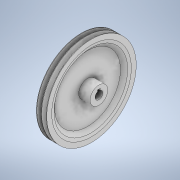
# Autodesk Inventor part: polia final
Saved by Autodesk Inventor 2022.1 (Build 261234020, 234B)
## iProperties
Created: 2023-10-20
Part Number: polia final
Material: Generic
Document SubType Name: Modeling
Designer: SENAI
Density: 1 g/cm^3
Appearance: Default
Author: SENAI
Autodesk Inventor part; units mm, degrees
ref_plane "YZ Plane" through (0, 0, 0) normal (1, 0, 0) x (0, 1, 0)
ref_plane "XZ Plane" through (0, 0, 0) normal (0, 1, 0) x (-1, 0, 0)
ref_plane "XY Plane" through (0, 0, 0) normal (0, 0, 1) x (1, 0, 0)
sketch "Sketch1" plane through (0, 0, 0) normal (0, 0, 1) x (1, 0, 0)
  line L0 (0, 0) -> (47, 0)
  line L1 (47, 10.25) -> (0, 10.25)
  line L2 (0, 10.25) -> (0, 17.75)
  line L3 (47, 10.25) -> (47, 23.25)
  line L4 (47, 23.25) -> (17, 23.25)
  line L5 (17, 23.25) -> (17, 86.75)
  line L6 (17, 86.75) -> (25.6776, 97.0916)
  line L7 (25.6776, 97.0916) -> (27.4678, 104.8887)
  line L8 (27.4678, 104.8887) -> (27.4678, 117.8887)
  line L9 (27.4678, 117.8887) -> (26.1178, 117.8887)
  line L10 (26.1178, 117.8887) -> (22.9803, 105.273)
  line L11 (22.9803, 105.273) -> (16.9803, 105.273)
  line L12 (16.9803, 105.273) -> (13.8419, 117.8885)
  line L13 (13.8419, 117.8885) -> (12.4919, 117.8885)
  line L14 (12.4919, 117.8885) -> (9.3536, 105.273)
  line L15 (9.3536, 105.273) -> (3.3536, 105.273)
  line L16 (0, 117.8885) -> (1.35, 117.8885)
  line L17 (1.35, 117.8885) -> (3.3536, 105.273)
  line L18 (0, 117.8885) -> (0, 103.8885)
  line L19 (0, 103.8885) -> (2.2376, 94.1421)
  line L20 (2.2376, 94.1421) -> (10.2376, 94.1421)
  line L21 (0, 17.75) -> (10.2376, 24.25)
  line L22 (10.2376, 94.1421) -> (10.2376, 24.25)
  dimension "d0" = 47
  dimension "d1" = 10.25
  dimension "d3" = 7.5
  dimension "d4" = 13
  dimension "d27" = 30
  dimension "d28" = 63.5
  dimension "d34" = 13.5
  dimension "d35" = 140
  dimension "d36" = 8
  dimension "d37" = 13
  dimension "d38" = 1.35
  dimension "d39" = 13
  dimension "d40" = 4.4875
  dimension "d41" = 6
  dimension "d42" = 13
  dimension "d43" = 103.97
  dimension "d44" = 1.35
  dimension "d47" = 13
  dimension "d48" = 6
  dimension "d49" = 103.97
  dimension "d51" = 1.35
  dimension "d52" = 14
  dimension "d53" = 10
  dimension "d54" = 167.07
  dimension "d55" = 8
  constraints: 46 end point, 9 horizontal, 6 vertical
  measures "d0" distance of L0.start L0.end
  measures "d1" distance of L0.end L1.start
  measures "d3" distance of L1.end L2.end
  measures "d4" distance of L1.start L3.end
  measures "d27" distance of L3.end L4.end
  measures "d28" distance of L4.end L5.end
  measures "d34" distance of L5.end L6.end
  measures "d35" angle of L5 L6
  measures "d36" distance of L6.end L7.end
  measures "d37" distance of L7.end L8.end
  measures "d38" distance of L8.end L9.end
  measures "d39" distance of L9.end L10.end
  measures "d40" distance from line of L8 L10.end
  measures "d41" distance of L10.end L11.end
  measures "d42" distance of L11.end L12.end
  measures "d43" angle of L12 L11
  measures "d44" distance of L12.end L13.end
  measures "d47" distance of L13.end L14.end
  measures "d48" distance of L14.end L15.end
  measures "d49" angle of L15 L14
  measures "d51" distance of L16.start L16.end
  measures "d52" distance of L16.start L18.end
  measures "d53" distance of L18.end L19.end
  measures "d54" angle of L19 L18
  measures "d55" distance of L19.end L20.end
revolve "Revolution1" add sketch "Sketch1" angle 360 about axis through (0, 0, 0) along (1, 0, 0)
sketch "Sketch2" plane through (0, 0, 0) normal (-1, 0, 0) x (0, 0, 1)
  circle A0 centre (0, 0) radius 17.75 projected
  line L0 (-3.5, 13.75) -> (3.5, 13.75)
  line L1 (3.5, 13.75) -> (3.5, 9.75)
  line L2 (3.5, 9.75) -> (-3.5, 9.75)
  line L3 (-3.5, 9.75) -> (-3.5, 13.75)
  dimension "d61" = 7
  dimension "d62" = 4
  constraints: 8 end point, 2 parallel, 1 horizontal, 1 perpendicular
  measures "d61" distance of L1.end L2.end
  measures "d62" distance of L0.end L1.end
extrude "Extrusion1" cut sketch "Sketch2" against normal blind 50 contours L0 L1 L2 L3
body "Solid1"
